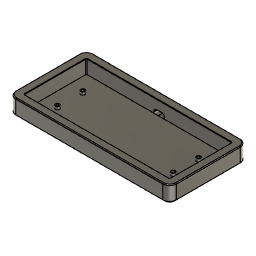
Boxy Bruce (Autodesk Fusion 360 design; units mm, degrees)
Autodesk Fusion 360 part; units mm, degrees
sketch "Outline Sketch" plane through (0, 0, 0) normal (0, 0, 1) x (1, 0, 0)
  line L0 (25.0077, 13.2259) -> (215.5077, 13.2259) construction
  line L1 (215.5077, 13.2259) -> (215.5077, 94.1884) construction
  line L2 (215.5077, 94.1884) -> (25.0077, 94.1884) construction
  line L3 (25.0077, 94.1884) -> (25.0077, 13.2259) construction
  line L4 (24.5077, 12.7259) -> (216.0077, 12.7259)
  line L5 (216.0077, 12.7259) -> (216.0077, 94.6884)
  line L6 (216.0077, 94.6884) -> (24.5077, 94.6884)
  line L7 (24.5077, 94.6884) -> (24.5077, 12.7259)
  line L8 (14.5077, 2.7259) -> (226.0077, 2.7259)
  line L9 (226.0077, 2.7259) -> (226.0077, 104.6884)
  line L10 (226.0077, 104.6884) -> (14.5077, 104.6884)
  line L11 (14.5077, 104.6884) -> (14.5077, 2.7259)
  dimension "d1" = 190.5
  dimension "d2" = 80.9625
  dimension "d3" = 0.5
  dimension "d4" = 10.5
  constraint horizontal L0
  constraint vertical L1
  constraint horizontal L2
  constraint vertical L3
  measures "d1" distance of L0.start L0.end
  measures "d2" distance of L0.start L2.end
extrude "Extrude1" add sketch "Outline Sketch" along normal blind 18.06
sketch "Angle Sketch" plane through (226.0077, 0, 0) normal (1, 0, 0) x (0, 1, 0)
  line L0 (2.7259, 0) -> (104.6884, 0)
  line L1 (104.6884, 0) -> (104.6884, 18.06)
  line L2 (104.6884, 18.06) -> (2.7259, 18.06)
  line L3 (2.7259, 18.06) -> (2.7259, 0)
  line L4 (2.7259, 18.06) -> (2.7259, -3.94) construction
  line L5 (2.7259, -3.94) -> (102.5888, -9.1736)
  line L6 (2.7259, -3.94) -> (102.7259, -3.94)
  dimension "d7" = 22
  dimension "d8" = 100
  dimension "d9" = 3
  constraint coincident L2.end L3.start
  constraint perpendicular L0 L4
  constraint horizontal L6
  measures "d7" distance of L2.end L4.end
  measures "d8" distance of L4.end L5.end
  measures "d9" angle of L5 L6
ref_plane "WorkPlane1" through (226.0077, 52.7259, -3.94) normal (0, 0, -1) x (0, 1, 0)
sketch "Bottom Sketch for Angle" plane through (0, 0, 0) normal (0, 0, -1) x (1, 0, 0)
  line L0 (24.5077, -94.6884) -> (24.5077, -12.7259)
  line L1 (24.5077, -12.7259) -> (216.0077, -12.7259)
  line L2 (216.0077, -12.7259) -> (216.0077, -94.6884)
  line L3 (216.0077, -94.6884) -> (24.5077, -94.6884)
  line L4 (14.5077, -2.7259) -> (14.5077, -104.6884)
  line L5 (14.5077, -104.6884) -> (226.0077, -104.6884)
  line L6 (226.0077, -104.6884) -> (226.0077, -2.7259)
  line L7 (226.0077, -2.7259) -> (14.5077, -2.7259)
  line L8 (226.0077, -104.6884) -> (14.5077, -104.6884)
  line L9 (14.5077, -104.6884) -> (14.5077, -2.7259)
  line L10 (14.5077, -2.7259) -> (226.0077, -2.7259)
  line L11 (226.0077, -2.7259) -> (226.0077, -104.6884)
  constraint horizontal L8
  constraint vertical L9
  constraint horizontal L10
  constraint vertical L11
  constraint coincident L4.start L7.end
  constraint coincident L5.end L6.start
extrude "Extrude2" add sketch "Bottom Sketch for Angle" along normal up to surface (3.94 mm away) contours L0 L1 L2 L3 | L4 L5 L6 L7 L8 L9 L10 L11
sketch "USB C Hole Internal Sketch" plane through (0, 94.6884, 0) normal (0, -1, 0) x (1, 0, 0)
  line L0 (24.5077, 0) -> (216.0077, 0)
  line L1 (216.0077, 0) -> (216.0077, 18.06)
  line L2 (216.0077, 18.06) -> (24.5077, 18.06)
  line L3 (24.5077, 18.06) -> (24.5077, 0)
  line L4 (120.2577, 0) -> (120.2577, 1.83) construction
  line L5 (124.9827, 3.66) -> (115.5327, 3.66)
  line L6 (115.5327, 3.66) -> (115.5327, 0)
  line L7 (115.5327, 0) -> (124.9827, 0)
  line L8 (124.9827, 0) -> (124.9827, 3.66)
  line L9 (124.9827, 3.66) -> (115.5327, 0) construction
  line L10 (115.5327, 3.66) -> (124.9827, 0) construction
  point P0 (120.2577, 1.83)
  dimension "d13" = 1.83
  dimension "d14" = 9.45
  dimension "d15" = 3.66
  constraint midpoint L0 L4.start
  constraint perpendicular L0 L4
  constraint horizontal L5
  constraint perpendicular L5 L6
  constraint parallel L5 L7
  constraint parallel L6 L8
  constraint coincident L9 P0
  constraint coincident L10 P0
  constraint coincident P0 L4.end
  measures "d13" distance of L4.start P0
  measures "d14" distance of L6.end L7.end
  measures "d15" distance of L5.end L6.end
extrude "Extrude3" cut sketch "USB C Hole Internal Sketch" against normal through all contours L0 L5 L6 L7 L8
fillet "Fillet1" radius 1.55 4 edges at (115.5327, 99.6884, 0) (115.5327, 99.6884, 3.66) (124.9827, 99.6884, 3.66) (124.9827, 99.6884, 0)
sketch "USB C Jut Sketch" plane through (0, 0, 0) normal (0, 0, 1) x (-1, 0, 0)
  line L0 (-123.4327, -94.6884) -> (-123.4327, -104.6884)
  line L1 (-123.4327, -104.6884) -> (-117.0827, -104.6884)
  line L2 (-117.0827, -104.6884) -> (-117.0827, -94.6884)
  line L3 (-117.0827, -94.6884) -> (-24.5077, -94.6884)
  line L4 (-24.5077, -94.6884) -> (-24.5077, -12.7259)
  line L5 (-24.5077, -12.7259) -> (-216.0077, -12.7259)
  line L6 (-216.0077, -12.7259) -> (-216.0077, -94.6884)
  line L7 (-216.0077, -94.6884) -> (-123.4327, -94.6884)
  line L8 (-117.0827, -94.6884) -> (-123.4327, -94.6884) construction
  line L9 (-125.7577, -99.6884) -> (-114.7577, -99.6884)
  line L10 (-114.7577, -99.6884) -> (-114.7577, -89.6884)
  line L11 (-114.7577, -89.6884) -> (-125.7577, -89.6884)
  line L12 (-125.7577, -89.6884) -> (-125.7577, -99.6884)
  line L13 (-125.7577, -99.6884) -> (-114.7577, -89.6884) construction
  line L14 (-114.7577, -99.6884) -> (-125.7577, -89.6884) construction
  point P0 (-120.2577, -94.6884)
  dimension "d19" = 11
  dimension "d20" = 10
  constraint coincident L2.end L3.start
  constraint coincident L0.start L7.end
  constraint horizontal L9
  constraint perpendicular L9 L10
  constraint parallel L9 L11
  constraint parallel L10 L12
  constraint coincident L13 P0
  constraint coincident L14 P0
  constraint midpoint L8 P0
  measures "d19" distance of L10.end L11.end
  measures "d20" distance of L9.start L11.end
extrude "Extrude4" cut sketch "USB C Jut Sketch" along normal blind 5.76 contours L0 L2 L3 L7 L9 L10 L11 L12 | L0 L7 L9 L12 | L2 L3 L9 L10
sketch "USB C Hole External Sketch" plane through (0, 104.6884, 0) normal (0, 1, 0) x (-1, 0, 0)
  line L0 (-117.0827, 0) -> (-123.4327, 0)
  arc A0 (-124.9827, 1.55) -> (-123.4327, 0) centre (-123.4327, 1.55) ccw
  line L1 (-124.9827, 1.55) -> (-124.9827, 2.11)
  arc A1 (-123.4327, 3.66) -> (-124.9827, 2.11) centre (-123.4327, 2.11) ccw
  line L2 (-123.4327, 3.66) -> (-117.0827, 3.66)
  arc A2 (-115.5327, 2.11) -> (-117.0827, 3.66) centre (-117.0827, 2.11) ccw
  line L3 (-115.5327, 2.11) -> (-115.5327, 1.55)
  arc A3 (-117.0827, 0) -> (-115.5327, 1.55) centre (-117.0827, 1.55) ccw
  line L4 (-14.5077, -3.94) -> (-14.5077, 18.06)
  line L5 (-14.5077, 18.06) -> (-226.0077, 18.06)
  line L6 (-226.0077, 18.06) -> (-226.0077, -3.94)
  line L7 (-226.0077, -3.94) -> (-14.5077, -3.94)
  line L8 (-124.9827, 1.83) -> (-115.5327, 1.83) construction
  line L9 (-120.2577, 0) -> (-120.2577, 3.66) construction
  line L10 (-113.2827, 5.91) -> (-127.2327, 5.91)
  line L11 (-127.2327, 5.91) -> (-127.2327, -2.25)
  line L12 (-127.2327, -2.25) -> (-113.2827, -2.25)
  line L13 (-113.2827, -2.25) -> (-113.2827, 5.91)
  line L14 (-113.2827, 5.91) -> (-127.2327, -2.25) construction
  line L15 (-127.2327, 5.91) -> (-113.2827, -2.25) construction
  point P0 (-120.2577, 1.83)
  dimension "d23" = 13.95
  dimension "d24" = 8.16
  constraint midpoint L1 L8.start
  constraint midpoint L3 L8.end
  constraint midpoint L0 L9.start
  constraint midpoint L2 L9.end
  constraint horizontal L10
  constraint perpendicular L10 L11
  constraint parallel L10 L12
  constraint parallel L11 L13
  constraint coincident L14 P0
  constraint coincident L15 P0
  constraint midpoint L8 P0
  measures "d23" distance of L11.end L12.end
  measures "d24" distance of L10.end L11.end
extrude "Extrude5" cut sketch "USB C Hole External Sketch" against normal up to surface (10 mm away) contours L10 L11 L12 L13
fillet "Fillet2" radius 3.8 4 edges at (127.2327, 99.6884, -2.25) (127.2327, 99.6884, 5.91) (113.2827, 99.6884, 5.91) (113.2827, 99.6884, -2.25)
chamfer "Chamfer1" distance 0.25 angle 45 8 edges at (120.2577, 104.6884, 5.91) (114.3957, 104.6884, 4.797) (113.2827, 104.6884, 1.83) (114.3957, 104.6884, -1.137) (120.2577, 104.6884, -2.25) (126.1197, 104.6884, -1.137) (127.2327, 104.6884, 1.83) (126.1197, 104.6884, 4.797)
fillet "Fillet3" radius 9 4 edges at (14.5077, 104.6884, 7.06) (14.5077, 2.7259, 7.06) (226.0077, 2.7259, 7.06) (226.0077, 104.6884, 7.06)
fillet "Fillet4" radius 1 4 edges at (24.5077, 94.6884, 9.03) (24.5077, 12.7259, 9.03) (216.0077, 12.7259, 9.03) (216.0077, 94.6884, 9.03)
fillet "Fillet6" radius 0.5 8 edges at (215.7148, 94.3955, 18.06) (216.0077, 53.7071, 18.06) (215.7148, 13.0188, 18.06) (120.2577, 12.7259, 18.06) (24.8006, 13.0188, 18.06) (24.5077, 53.7071, 18.06) (24.8006, 94.3955, 18.06) (120.2577, 94.6884, 18.06)
chamfer "Chamfer3" distance 3 angle 45 8 edges at (120.2577, 2.7259, -3.94) (223.3716, 5.3619, -3.94) (226.0077, 53.7071, -3.94) (223.3716, 102.0524, -3.94) (120.2577, 104.6884, -3.94) (17.1437, 102.0524, -3.94) (14.5077, 53.7071, -3.94) (17.1437, 5.3619, -3.94)
fillet "Fillet5" radius 1 8 edges at (223.3716, 5.3619, 18.06) (226.0077, 53.7071, 18.06) (223.3716, 102.0524, 18.06) (120.2577, 104.6884, 18.06) (17.1437, 102.0524, 18.06) (14.5077, 53.7071, 18.06) (17.1437, 5.3619, 18.06) (120.2577, 2.7259, 18.06)
sketch "Screw Post Sketch" plane through (0, 0, 0) normal (0, 0, 1) x (-1, 0, 0)
  arc A0 (-216.0077, -93.6884) -> (-215.0077, -94.6884) centre (-215.0077, -93.6884) ccw
  line L0 (-215.0077, -94.6884) -> (-126.9022, -94.6884)
  line L1 (-126.9022, -94.6884) -> (-113.6132, -94.6884)
  line L2 (-113.6132, -94.6884) -> (-25.5077, -94.6884)
  arc A1 (-25.5077, -94.6884) -> (-24.5077, -93.6884) centre (-25.5077, -93.6884) ccw
  line L3 (-24.5077, -93.6884) -> (-24.5077, -13.7259)
  arc A2 (-24.5077, -13.7259) -> (-25.5077, -12.7259) centre (-25.5077, -13.7259) ccw
  line L4 (-25.5077, -12.7259) -> (-215.0077, -12.7259)
  arc A3 (-215.0077, -12.7259) -> (-216.0077, -13.7259) centre (-215.0077, -13.7259) ccw
  line L5 (-216.0077, -13.7259) -> (-216.0077, -93.6884)
  line L6 (-24.5077, -94.6884) -> (-216.0077, -94.6884) construction
  line L7 (-216.0077, -94.6884) -> (-216.0077, -12.7259) construction
  line L8 (-216.0077, -12.7259) -> (-24.5077, -12.7259) construction
  line L9 (-24.5077, -12.7259) -> (-24.5077, -94.6884) construction
  line L10 (-25.0077, -94.1884) -> (-215.5077, -94.1884)
  line L11 (-215.5077, -94.1884) -> (-215.5077, -13.2259)
  line L12 (-215.5077, -13.2259) -> (-25.0077, -13.2259)
  line L13 (-25.0077, -13.2259) -> (-25.0077, -94.1884)
  circle A4 centre (-44.0577, -70.3759) radius 2.75
  circle A5 centre (-196.4577, -70.3759) radius 2.75
  circle A6 centre (-196.4577, -37.0384) radius 2.75
  circle A7 centre (-44.0577, -37.0384) radius 2.75
  dimension "d36" = 191.5
  dimension "d37" = 81.9625
  dimension "d38" = 0.5
  dimension "d39" = 5.5
  dimension "d40" = 19.05
  dimension "d41" = 23.8125
  dimension "d42" = 19.05
  dimension "d43" = 23.8125
  dimension "d44" = 19.05
  dimension "d45" = 23.8125
  dimension "d46" = 19.05
  dimension "d47" = 23.8125
  constraint horizontal L6
  constraint vertical L7
  constraint horizontal L8
  constraint vertical L9
  constraint equal A4 A5
  constraint equal A4 A7
  constraint equal A4 A6
  measures "d36" distance of L6.start L6.end
  measures "d37" distance of L6.start L8.end
  measures "d39" diameter of A4
  measures "d40" distance of L13 A4.centre
  measures "d41" distance of L10 A4.centre
  measures "d42" distance of L11 A5.centre
  measures "d43" distance of L10 A5.centre
  measures "d44" distance of L11 A6.centre
  measures "d45" distance of L12 A6.centre
  measures "d46" distance of L13 A7.centre
  measures "d47" distance of L12 A7.centre
extrude "Extrude6" add sketch "Screw Post Sketch" along normal blind 3.46 contours A4 | A5 | A6 | A7
hole "Hole1" at (44.0577, 70.3759, 3.46) direction (0, 0, -1) diameter 3.2 depth 4 tip angle 180
hole "Hole2" at (44.0577, 37.0384, 3.46) direction (0, 0, -1) diameter 3.2 depth 4 tip angle 180
hole "Hole3" at (196.4577, 70.3759, 3.46) direction (0, 0, -1) diameter 3.2 depth 4 tip angle 180
hole "Hole4" at (196.4577, 37.0384, 3.46) direction (0, 0, -1) diameter 3.2 depth 4 tip angle 180
move_body "Move1" [rolled back] rotate angle -3
equation "d1 = 19.05 mm * 10"
equation "d2 = 19.05 mm * 4.25"
equation "d13 = ( 3.66 / 2 ) * 1 mm"
equation "d21 = 3.66 mm + 1.6 mm + 0.5 mm"
equation "d36 = 19.05 mm * 10 + 1 mm"
equation "d37 = 19.05 mm * 4.25 + 1 mm"
equation "d41 = 19.05 mm * 1.25"
equation "d42 = d40"
equation "d43 = d41"
equation "d44 = d40"
equation "d45 = d41"
equation "d46 = d40"
equation "d47 = d41"
